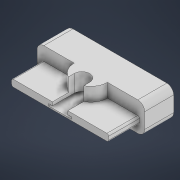
# Autodesk Inventor part: syringe_sledge_fitter
Saved by Autodesk Inventor 2022 (Build 260153000, 153)
## iProperties
Created: 2023-04-24
Part Number: syringe_sledge_fitter
Material: Generic
Document SubType Name: Modeling
Designer: Jakob Saugbjerg
Density: 1 g/cm^3
Appearance: Default
Author: Jakob Saugbjerg
Autodesk Inventor part; units mm, degrees
ref_plane "YZ Plane" through (0, 0, 0) normal (1, 0, 0) x (0, 1, 0)
ref_plane "XZ Plane" through (0, 0, 0) normal (0, 1, 0) x (-1, 0, 0)
ref_plane "XY Plane" through (0, 0, 0) normal (0, 0, 1) x (1, 0, 0)
sketch "Sketch1" plane through (0, 0, 0) normal (0, 0, 1) x (1, 0, 0)
  line L0 (0, 0) -> (63, 0)
  line L1 (63, 0) -> (63, 17)
  line L2 (63, 17) -> (0, 17)
  line L3 (0, 17) -> (0, 0)
  dimension "d0" = 63
  dimension "d1" = 17
  constraints: 8 end point, 2 parallel, 1 horizontal, 1 perpendicular
  measures "d0" distance of L2.end L1.end
  measures "d1" distance of L1.end L0.end
extrude "Extrusion1" add sketch "Sketch1" along normal blind 35
sketch "Sketch10" plane through (0, 0, 0) normal (0, 0, -1) x (-1, 0, 0)
  line L0 (-19.9115, 8.8287) -> (-18.0318, 8.8287)
  line L1 (-18.0318, 8.8287) -> (-18.0318, 8.3965)
  spline S0 degree 2 poles (-18.0318, 8.3965) (-18.2344, 8.2063) (-18.595, 7.8531) (-18.7679, 7.6629) knots 0 0 0 1 2 2 2
  spline S1 degree 2 poles (-18.7679, 7.6629) (-19.1162, 7.28) (-19.3706, 6.8206) (-19.3706, 6.5761) knots 0 0 0 1 2 2 2
  spline S2 degree 2 poles (-19.3706, 6.5761) (-19.3706, 6.4476) (-19.2915, 6.255) (-19.2199, 6.1932) knots 0 0 0 1 2 2 2
  spline S3 degree 2 poles (-19.2199, 6.1932) (-19.1483, 6.1315) (-18.9606, 6.0697) (-18.8469, 6.0697) knots 0 0 0 1 2 2 2
  spline S4 degree 2 poles (-18.8469, 6.0697) (-18.7383, 6.0697) (-18.5159, 6.1241) (-18.4147, 6.1661) knots 0 0 0 1 2 2 2
  spline S5 degree 2 poles (-18.4147, 6.1661) (-18.3282, 6.2006) (-18.1677, 6.2994) (-18.1183, 6.334) knots 0 0 0 1 2 2 2
  line L2 (-18.1183, 6.334) -> (-18.096, 6.334)
  line L3 (-18.096, 6.334) -> (-18.096, 5.8993)
  spline S6 degree 2 poles (-18.096, 5.8993) (-18.222, 5.8375) (-18.674, 5.7165) (-18.8766, 5.7165) knots 0 0 0 1 2 2 2
  spline S7 degree 2 poles (-18.8766, 5.7165) (-19.3039, 5.7165) (-19.7855, 6.1685) (-19.7855, 6.5539) knots 0 0 0 1 2 2 2
  spline S8 degree 2 poles (-19.7855, 6.5539) (-19.7855, 6.7342) (-19.7016, 7.0355) (-19.6275, 7.1639) knots 0 0 0 1 2 2 2
  spline S9 degree 2 poles (-19.6275, 7.1639) (-19.5534, 7.2973) (-19.3385, 7.5591) (-19.2199, 7.6851) knots 0 0 0 1 2 2 2
  spline S10 degree 2 poles (-19.2199, 7.6851) (-19.0272, 7.8951) (-18.5555, 8.3446) (-18.4147, 8.4755) knots 0 0 0 1 2 2 2
  line L4 (-18.4147, 8.4755) -> (-19.9115, 8.4755)
  line L5 (-19.9115, 8.4755) -> (-19.9115, 8.8287)
  line L6 (-24.2785, 8.8287) -> (-24.2785, 7.5048)
  spline S11 degree 2 poles (-24.2785, 7.5048) (-24.2785, 7.3467) (-24.2538, 7.0775) (-24.2143, 7.0034) knots 0 0 0 1 2 2 2
  spline S12 degree 2 poles (-24.2143, 7.0034) (-24.1748, 6.9219) (-24.0241, 6.8428) (-23.8932, 6.8428) knots 0 0 0 1 2 2 2
  spline S13 degree 2 poles (-23.8932, 6.8428) (-23.7746, 6.8428) (-23.5029, 6.9886) (-23.3597, 7.1269) knots 0 0 0 1 2 2 2
  spline S14 degree 2 poles (-23.3597, 7.1269) (-23.3621, 7.1615) (-23.3671, 7.2578) (-23.3671, 7.322) knots 0 0 0 1 2 2 2
  line L7 (-23.3671, 7.322) -> (-23.3671, 8.8287)
  line L8 (-23.3671, 8.8287) -> (-22.9817, 8.8287)
  line L9 (-22.9817, 8.8287) -> (-22.9817, 7.5048)
  spline S15 degree 2 poles (-22.9817, 7.5048) (-22.9817, 7.3467) (-22.957, 7.0775) (-22.9175, 7.0034) knots 0 0 0 1 2 2 2
  spline S16 degree 2 poles (-22.9175, 7.0034) (-22.878, 6.9219) (-22.7273, 6.8428) (-22.5964, 6.8428) knots 0 0 0 1 2 2 2
  spline S17 degree 2 poles (-22.5964, 6.8428) (-22.4729, 6.8428) (-22.1987, 6.9985) (-22.0703, 7.1195) knots 0 0 0 1 2 2 2
  line L10 (-22.0703, 7.1195) -> (-22.0703, 8.8287)
  line L11 (-22.0703, 8.8287) -> (-21.685, 8.8287)
  line L12 (-21.685, 8.8287) -> (-21.685, 6.5415)
  line L13 (-21.685, 6.5415) -> (-22.0703, 6.5415)
  line L14 (-22.0703, 6.5415) -> (-22.0703, 6.7934)
  spline S18 degree 2 poles (-22.0703, 6.7934) (-22.221, 6.6428) (-22.5174, 6.4773) (-22.6952, 6.4773) knots 0 0 0 1 2 2 2
  spline S19 degree 2 poles (-22.6952, 6.4773) (-22.8978, 6.4773) (-23.2114, 6.6625) (-23.293, 6.8725) knots 0 0 0 1 2 2 2
  spline S20 degree 2 poles (-23.293, 6.8725) (-23.4683, 6.6774) (-23.7993, 6.4773) (-23.992, 6.4773) knots 0 0 0 1 2 2 2
  spline S21 degree 2 poles (-23.992, 6.4773) (-24.1402, 6.4773) (-24.3822, 6.5687) (-24.4712, 6.6724) knots 0 0 0 1 2 2 2
  spline S22 degree 2 poles (-24.4712, 6.6724) (-24.5625, 6.7762) (-24.6638, 7.0874) (-24.6638, 7.322) knots 0 0 0 1 2 2 2
  line L15 (-24.6638, 7.322) -> (-24.6638, 8.8287)
  line L16 (-24.6638, 8.8287) -> (-24.2785, 8.8287)
  line L17 (-27.0005, 8.8287) -> (-25.2344, 8.8287)
  line L18 (-25.2344, 8.8287) -> (-25.2344, 5.7807)
  line L19 (-25.2344, 5.7807) -> (-25.6395, 5.7807)
  line L20 (-25.6395, 5.7807) -> (-25.6395, 8.4681)
  line L21 (-25.6395, 8.4681) -> (-27.0005, 8.4681)
  line L22 (-27.0005, 8.4681) -> (-27.0005, 8.8287)
  spline S23 degree 2 poles (-29.2161, 8.8831) (-28.9863, 8.8831) (-28.5887, 8.7596) (-28.4578, 8.6904) knots 0 0 0 1 2 2 2
  line L23 (-28.4578, 8.6904) -> (-28.4578, 8.2582)
  line L24 (-28.4578, 8.2582) -> (-28.4775, 8.2582)
  spline S24 degree 2 poles (-28.4775, 8.2582) (-28.5269, 8.2977) (-28.6603, 8.3915) (-28.7715, 8.4434) knots 0 0 0 1 2 2 2
  spline S25 degree 2 poles (-28.7715, 8.4434) (-28.8678, 8.4903) (-29.1049, 8.5595) (-29.2309, 8.5595) knots 0 0 0 1 2 2 2
  spline S26 degree 2 poles (-29.2309, 8.5595) (-29.3223, 8.5595) (-29.5322, 8.5175) (-29.5816, 8.4829) knots 0 0 0 1 2 2 2
  spline S27 degree 2 poles (-29.5816, 8.4829) (-29.6533, 8.436) (-29.7175, 8.3298) (-29.7175, 8.2211) knots 0 0 0 1 2 2 2
  spline S28 degree 2 poles (-29.7175, 8.2211) (-29.7175, 8.0853) (-29.5693, 7.9445) (-29.3791, 7.8975) knots 0 0 0 1 2 2 2
  spline S29 degree 2 poles (-29.3791, 7.8975) (-29.305, 7.8803) (-29.0679, 7.8309) (-28.9666, 7.8037) knots 0 0 0 1 2 2 2
  spline S30 degree 2 poles (-28.9666, 7.8037) (-28.7048, 7.7271) (-28.4676, 7.4109) (-28.4676, 7.1862) knots 0 0 0 1 2 2 2
  spline S31 degree 2 poles (-28.4676, 7.1862) (-28.4676, 6.875) (-28.9345, 6.4872) (-29.3198, 6.4872) knots 0 0 0 1 2 2 2
  spline S32 degree 2 poles (-29.3198, 6.4872) (-29.51, 6.4872) (-29.8953, 6.581) (-30.0262, 6.6527) knots 0 0 0 1 2 2 2
  line L25 (-30.0262, 6.6527) -> (-30.0262, 7.0651)
  line L26 (-30.0262, 7.0651) -> (-30.0065, 7.0651)
  spline S33 degree 2 poles (-30.0065, 7.0651) (-29.8583, 6.9466) (-29.4976, 6.8107) (-29.3124, 6.8107) knots 0 0 0 1 2 2 2
  spline S34 degree 2 poles (-29.3124, 6.8107) (-29.1222, 6.8107) (-28.8604, 6.9713) (-28.8604, 7.1318) knots 0 0 0 1 2 2 2
  spline S35 degree 2 poles (-28.8604, 7.1318) (-28.8604, 7.2776) (-29.016, 7.4184) (-29.1889, 7.4628) knots 0 0 0 1 2 2 2
  spline S36 degree 2 poles (-29.1889, 7.4628) (-29.2729, 7.485) (-29.4853, 7.5295) (-29.6014, 7.5567) knots 0 0 0 1 2 2 2
  spline S37 degree 2 poles (-29.6014, 7.5567) (-29.8533, 7.6209) (-30.1102, 7.9148) (-30.1102, 8.1692) knots 0 0 0 1 2 2 2
  spline S38 degree 2 poles (-30.1102, 8.1692) (-30.1102, 8.3174) (-29.9941, 8.5793) (-29.8805, 8.6756) knots 0 0 0 1 2 2 2
  spline S39 degree 2 poles (-29.8805, 8.6756) (-29.7595, 8.7769) (-29.4507, 8.8831) (-29.2161, 8.8831) knots 0 0 0 1 2 2 2
  line L27 (-32.2641, 6.5415) -> (-31.034, 9.671)
  line L28 (-31.034, 9.671) -> (-30.6215, 9.671)
  line L29 (-30.6215, 9.671) -> (-31.0315, 8.7176)
  line L30 (-31.0315, 8.7176) -> (-30.2016, 6.5415)
  line L31 (-30.2016, 6.5415) -> (-30.6166, 6.5415)
  line L32 (-30.6166, 6.5415) -> (-31.2415, 8.2359)
  line L33 (-31.2415, 8.2359) -> (-31.8639, 6.5415)
  line L34 (-31.8639, 6.5415) -> (-32.2641, 6.5415)
  line L35 (-33.7683, 6.954) -> (-33.7485, 6.954)
  spline S40 degree 2 poles (-33.7485, 6.954) (-33.7041, 6.9416) (-33.6077, 6.9367) (-33.5411, 6.9367) knots 0 0 0 1 2 2 2
  spline S41 degree 2 poles (-33.5411, 6.9367) (-33.3854, 6.9367) (-33.0792, 7.0726) (-32.9408, 7.2059) knots 0 0 0 1 2 2 2
  line L36 (-32.9408, 7.2059) -> (-32.9408, 8.8287)
  line L37 (-32.9408, 8.8287) -> (-32.5555, 8.8287)
  line L38 (-32.5555, 8.8287) -> (-32.5555, 6.5415)
  line L39 (-32.5555, 6.5415) -> (-32.9408, 6.5415)
  line L40 (-32.9408, 6.5415) -> (-32.9408, 6.8824)
  spline S42 degree 2 poles (-32.9408, 6.8824) (-33.1508, 6.6946) (-33.4645, 6.5415) (-33.6127, 6.5415) knots 0 0 0 1 2 2 2
  spline S43 degree 2 poles (-33.6127, 6.5415) (-33.672, 6.5415) (-33.7312, 6.5464) (-33.7683, 6.5539) knots 0 0 0 1 2 2 2
  line L41 (-33.7683, 6.5539) -> (-33.7683, 6.954)
  line L42 (-34.4599, 8.8287) -> (-34.0746, 8.8287)
  line L43 (-34.0746, 8.8287) -> (-34.0746, 6.5415)
  line L44 (-34.0746, 6.5415) -> (-34.4599, 6.5415)
  line L45 (-34.4599, 6.5415) -> (-34.4599, 8.8287)
  line L46 (-34.4871, 6.1611) -> (-34.0499, 6.1611)
  line L47 (-34.0499, 6.1611) -> (-34.0499, 5.761)
  line L48 (-34.0499, 5.761) -> (-34.4871, 5.761)
  line L49 (-34.4871, 5.761) -> (-34.4871, 6.1611)
  line L50 (-36.8212, 8.8287) -> (-36.4359, 8.8287)
  line L51 (-36.4359, 8.8287) -> (-36.4359, 7.5246)
  spline S44 degree 2 poles (-36.4359, 7.5246) (-36.4359, 7.3665) (-36.4063, 7.0948) (-36.3618, 7.0133) knots 0 0 0 1 2 2 2
  spline S45 degree 2 poles (-36.3618, 7.0133) (-36.3149, 6.9268) (-36.1469, 6.8428) (-36.0037, 6.8428) knots 0 0 0 1 2 2 2
  spline S46 degree 2 poles (-36.0037, 6.8428) (-35.8604, 6.8428) (-35.5566, 6.996) (-35.4109, 7.1195) knots 0 0 0 1 2 2 2
  line L52 (-35.4109, 7.1195) -> (-35.4109, 8.8287)
  line L53 (-35.4109, 8.8287) -> (-35.0255, 8.8287)
  line L54 (-35.0255, 8.8287) -> (-35.0255, 6.5415)
  line L55 (-35.0255, 6.5415) -> (-35.4109, 6.5415)
  line L56 (-35.4109, 6.5415) -> (-35.4109, 6.7959)
  spline S47 degree 2 poles (-35.4109, 6.7959) (-35.5838, 6.6403) (-35.9172, 6.4773) (-36.1049, 6.4773) knots 0 0 0 1 2 2 2
  spline S48 degree 2 poles (-36.1049, 6.4773) (-36.4409, 6.4773) (-36.8212, 6.9219) (-36.8212, 7.3443) knots 0 0 0 1 2 2 2
  line L57 (-36.8212, 7.3443) -> (-36.8212, 8.8287)
  spline S49 degree 2 poles (-37.4437, 9.1943) (-37.4832, 9.2116) (-37.6339, 9.2659) (-37.7302, 9.2882) knots 0 0 0 1 2 2 2
  spline S50 degree 2 poles (-37.7302, 9.2882) (-37.8364, 9.3153) (-38.0167, 9.3474) (-38.1229, 9.3474) knots 0 0 0 1 2 2 2
  spline S51 degree 2 poles (-38.1229, 9.3474) (-38.3008, 9.3474) (-38.5478, 9.2536) (-38.6169, 9.1696) knots 0 0 0 1 2 2 2
  spline S52 degree 2 poles (-38.6169, 9.1696) (-38.6836, 9.0856) (-38.7355, 8.8658) (-38.7355, 8.725) knots 0 0 0 1 2 2 2
  line L58 (-38.7355, 8.725) -> (-38.7355, 8.5249)
  spline S53 degree 2 poles (-38.7355, 8.5249) (-38.5799, 8.6608) (-38.281, 8.7892) (-38.0562, 8.7892) knots 0 0 0 1 2 2 2
  spline S54 degree 2 poles (-38.0562, 8.7892) (-37.666, 8.7892) (-37.2041, 8.2088) (-37.2041, 7.6629) knots 0 0 0 1 2 2 2
  spline S55 degree 2 poles (-37.2041, 7.6629) (-37.2041, 7.3788) (-37.3646, 6.9392) (-37.498, 6.7836) knots 0 0 0 1 2 2 2
  spline S56 degree 2 poles (-37.498, 6.7836) (-37.6265, 6.6378) (-37.9797, 6.4773) (-38.1674, 6.4773) knots 0 0 0 1 2 2 2
  spline S57 degree 2 poles (-38.1674, 6.4773) (-38.3452, 6.4773) (-38.6046, 6.5613) (-38.7355, 6.6378) knots 0 0 0 1 2 2 2
  line L59 (-38.7355, 6.6378) -> (-38.7577, 6.5415)
  line L60 (-38.7577, 6.5415) -> (-39.1208, 6.5415)
  line L61 (-39.1208, 6.5415) -> (-39.1208, 8.5669)
  spline S58 degree 2 poles (-39.1208, 8.5669) (-39.1208, 9.1498) (-38.6145, 9.6932) (-38.0933, 9.6932) knots 0 0 0 1 2 2 2
  spline S59 degree 2 poles (-38.0933, 9.6932) (-37.9253, 9.6932) (-37.5746, 9.6389) (-37.4239, 9.5944) knots 0 0 0 1 2 2 2
  line L62 (-37.4239, 9.5944) -> (-37.4239, 9.1943)
  line L63 (-37.4239, 9.1943) -> (-37.4437, 9.1943)
  line L64 (-38.7355, 8.2088) -> (-38.7355, 6.9515)
  spline S60 degree 2 poles (-38.7355, 6.9515) (-38.5922, 6.8824) (-38.3502, 6.8231) (-38.2291, 6.8231) knots 0 0 0 1 2 2 2
  spline S61 degree 2 poles (-38.2291, 6.8231) (-37.9377, 6.8231) (-37.6018, 7.2529) (-37.6018, 7.6555) knots 0 0 0 1 2 2 2
  spline S62 degree 2 poles (-37.6018, 7.6555) (-37.6018, 8.0359) (-37.8562, 8.4335) (-38.1427, 8.4335) knots 0 0 0 1 2 2 2
  spline S63 degree 2 poles (-38.1427, 8.4335) (-38.2934, 8.4335) (-38.6095, 8.315) (-38.7355, 8.2088) knots 0 0 0 1 2 2 2
  spline S64 degree 2 poles (-40.672, 8.8806) (-40.1237, 8.8806) (-39.521, 8.2656) (-39.521, 7.6975) knots 0 0 0 1 2 2 2
  spline S65 degree 2 poles (-39.521, 7.6975) (-39.521, 7.1392) (-40.1064, 6.4773) (-40.5781, 6.4773) knots 0 0 0 1 2 2 2
  spline S66 degree 2 poles (-40.5781, 6.4773) (-40.7906, 6.4773) (-41.1191, 6.6008) (-41.2401, 6.7317) knots 0 0 0 1 2 2 2
  spline S67 degree 2 poles (-41.2401, 6.7317) (-41.3636, 6.8626) (-41.4945, 7.2405) (-41.4945, 7.5147) knots 0 0 0 1 2 2 2
  line L65 (-41.4945, 7.5147) -> (-41.4945, 7.7246)
  line L66 (-41.4945, 7.7246) -> (-39.9112, 7.7246)
  spline S68 degree 2 poles (-39.9112, 7.7246) (-39.9112, 8.1223) (-40.3114, 8.5447) (-40.6671, 8.5447) knots 0 0 0 1 2 2 2
  spline S69 degree 2 poles (-40.6671, 8.5447) (-40.793, 8.5447) (-41.0376, 8.4879) (-41.1364, 8.4434) knots 0 0 0 1 2 2 2
  spline S70 degree 2 poles (-41.1364, 8.4434) (-41.2401, 8.394) (-41.3834, 8.3076) (-41.4303, 8.268) knots 0 0 0 1 2 2 2
  line L67 (-41.4303, 8.268) -> (-41.4525, 8.268)
  line L68 (-41.4525, 8.268) -> (-41.4525, 8.6879)
  spline S71 degree 2 poles (-41.4525, 8.6879) (-41.3858, 8.7151) (-41.1833, 8.7942) (-41.1042, 8.8164) knots 0 0 0 1 2 2 2
  spline S72 degree 2 poles (-41.1042, 8.8164) (-40.9931, 8.8485) (-40.8103, 8.8806) (-40.672, 8.8806) knots 0 0 0 1 2 2 2
  spline S73 degree 2 poles (-41.1191, 7.4307) (-41.1141, 7.2751) (-41.0499, 7.0479) (-40.9882, 6.9713) knots 0 0 0 1 2 2 2
  spline S74 degree 2 poles (-40.9882, 6.9713) (-40.9215, 6.8848) (-40.7115, 6.7934) (-40.5559, 6.7934) knots 0 0 0 1 2 2 2
  spline S75 degree 2 poles (-40.5559, 6.7934) (-40.4028, 6.7934) (-40.1879, 6.8848) (-40.099, 6.9738) knots 0 0 0 1 2 2 2
  spline S76 degree 2 poles (-40.099, 6.9738) (-40.0125, 7.0651) (-39.9236, 7.285) (-39.9112, 7.4307) knots 0 0 0 1 2 2 2
  line L69 (-39.9112, 7.4307) -> (-41.1191, 7.4307)
  point P0 (0, 0)
  point P1 (-17.8095, 5.7165)
  dimension "d3" = 0
  constraints: 1 other
emboss "Emboss1" sketch "Sketch10" operation cut depth 1 direction (0, 0, 1)
sketch "Sketch15" plane through (0, 0, 35) normal (0, 0, 1) x (1, 0, 0)
  line L0 (0, 17) -> (0, 0) projected
  line L1 (0, 0) -> (0, 5)
  line L2 (63, 0) -> (63, 17) projected
  line L3 (0, 5) -> (63, 5)
  line L4 (63, 5) -> (63, 0)
  line L5 (63, 0) -> (0, 0)
  line L6 (0, 0) -> (0, 5)
  line L7 (63, 17) -> (0, 17) projected
  line L8 (63, 17) -> (0, 17)
  line L9 (0, 17) -> (0, 9)
  line L10 (0, 9) -> (63, 9)
  line L11 (63, 9) -> (63, 17)
  dimension "d67" = 5
  dimension "d68" = 8
  constraints: 18 end point, 4 parallel, 2 horizontal, 2 perpendicular, 2 point on line
  measures "d67" distance of L0.end L1.end
  measures "d68" distance of L9.end L8.end
extrude "Extrusion12" cut sketch "Sketch15" against normal blind 18 contours L7 L2 L10 L0 | L3 L2 L5 L0
sketch "Sketch16" plane through (0, 9, 35) normal (0, 1, 0) x (1, 0, 0)
  line L0 (0, 0) -> (63, 0) projected
  line L1 (31.5, 0) -> (31.5, 12.75)
  circle A0 centre (31.5, 12.75) radius 4.5
  line L2 (27, 12.75) -> (36, 12.75)
  line L3 (36, 12.75) -> (36, 0)
  line L4 (36, 0) -> (27, 0)
  line L5 (27, 0) -> (27, 12.75)
  point P0 (0, 35)
  dimension "d88" = 12.75
  dimension "d89" = 9
  constraints: 10 end point, 2 parallel, 2 point on circle, 1 centre point, 1 coincident, 1 horizontal, 1 midpoint, 1 perpendicular, 1 vertical
  measures "d88" distance of L1.start L1.end
  measures "d89" diameter of A0
extrude "Extrusion13" cut sketch "Sketch16" against normal blind 2
sketch "Sketch17" plane through (0, 7, 35) normal (0, 1, 0) x (1, 0, 0)
  arc A0 (36, 12.75) -> (27, 12.75) centre (31.5, 12.75) ccw projected
  circle A1 centre (31.5, 12.75) radius 4.5
  circle A2 centre (31.5, 12.75) radius 6.7
  line L0 (24.8, 12.75) -> (38.2, 12.75)
  line L1 (38.2, 12.75) -> (38.2, 0)
  line L2 (38.2, 0) -> (24.8, 0)
  line L3 (24.8, 0) -> (24.8, 12.75)
  point P0 (0, 35)
  point P1 (31.5, 9.5)
  dimension "d90" = 13.4
  constraints: 8 end point, 2 centre point, 2 coincident, 2 parallel, 2 point on circle, 1 perpendicular
  measures "d90" diameter of A2
extrude "Extrusion14" cut sketch "Sketch17" against normal blind 1.2
sketch "Sketch18" plane through (0, 0, 35) normal (0, 0, 1) x (1, 0, 0)
  line L0 (0, 5) -> (63, 5) projected
  line L1 (3.1, 9) -> (59.9, 9)
  line L2 (59.9, 9) -> (59.9, 5)
  line L3 (59.9, 5) -> (3.1, 5)
  line L4 (3.1, 5) -> (3.1, 9)
  line L5 (3.1, 9) -> (59.9, 5) construction
  line L6 (59.9, 9) -> (3.1, 5) construction
  line L7 (63, 9) -> (0, 9) projected
  line L8 (59.9, 5) -> (63, 5)
  line L9 (63, 5) -> (63, 9)
  line L10 (63, 9) -> (59.9, 9)
  line L11 (59.9, 9) -> (59.9, 5)
  line L12 (0, 17) -> (0, 0) projected
  line L13 (3.1, 5) -> (0, 5)
  line L14 (0, 5) -> (0, 9)
  line L15 (0, 9) -> (3.1, 9)
  line L16 (3.1, 9) -> (3.1, 5)
  point P0 (31.5, 7)
  point P1 (37.25, 7)
  point P2 (3.1, 5)
  dimension "d78" = 56.8
  constraints: 26 end point, 5 parallel, 3 horizontal, 3 point on line, 2 midpoint, 2 perpendicular, 1 vertical, 4 other
  measures "d78" distance of L2.end L3.end
extrude "Extrusion15" cut sketch "Sketch18" against normal blind 18 contours L12 L7 L4 L0 | L2 L7 L9 L0
fillet "Fillet6" radius 1 4 edges at (3.1, 9, 26) (3.1, 5, 26) (59.9, 5, 26) (59.9, 9, 26)
fillet "Fillet7" radius 4 4 edges at (63, 17, 8.5) (63, 0, 8.5) (0, 0, 8.5) (0, 17, 8.5)
sketch "Sketch19" plane through (31.5, 9, 25.5) normal (0, 1, 0) x (1, 0, 0)
  line L0 (31.5, 8.5) -> (-31.5, 8.5) projected
  circle A0 centre (0, 8.5) radius 9.75
  arc A1 (4.5, 3.25) -> (-4.5, 3.25) centre (0, 3.25) ccw projected
  circle A2 centre (0, 3.25) radius 4.5
  line L1 (4.5, 3.25) -> (4.5, -9.5) projected
  line L2 (4.5, 3.25) -> (-4.5, 3.25)
  line L3 (-4.5, 3.25) -> (-4.5, -9.5)
  line L4 (-4.5, -9.5) -> (4.5, -9.5)
  line L5 (4.5, -9.5) -> (4.5, 3.25)
  point P0 (-31.5, 25.5)
  point P1 (27.4, 8.5)
  point P2 (-27.4, 8.5)
  point P3 (0, 0)
  point P4 (9.75, 8.5)
  point P5 (-9.75, 8.5)
  point P6 (-4.5, -0.1494)
  point P7 (4.5, -0.1494)
  dimension "d84" = 19.5
  constraints: 8 end point, 2 parallel, 2 perpendicular, 1 centre point, 1 coincident, 1 horizontal alignment, 1 midpoint, 2 other
  measures "d84" diameter of A0
extrude "Extrusion16" add sketch "Sketch19" along normal blind 8 contours A0 L1 A1 L3 L0 | L0 A0
body "Solid1"
